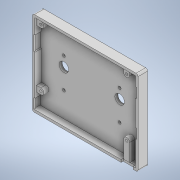
# Autodesk Inventor part: jetson_din_connector
Saved by Autodesk Inventor 2021 (Build 250183000, 183)
## iProperties
Created: 2020-10-27
Part Number: jetson_din_connector
Material: Generic
Document SubType Name: Modeling
Designer: Mateusz
Density: 1 g/cm^3
Appearance: Default
Author: Mateusz
Autodesk Inventor part; units mm, degrees
ref_plane "YZ Plane" through (0, 0, 0) normal (1, 0, 0) x (0, 1, 0)
ref_plane "XZ Plane" through (0, 0, 0) normal (0, 1, 0) x (-1, 0, 0)
ref_plane "Work Plane1" through (95.4, -17, 0) normal (0, 0, -1) x (-1, 0, 0)
sketch "Sketch1" plane through (95.4, -17, 0) normal (0, 0, -1) x (-1, 0, 0)
  line L0 (0, 79) -> (98.8, 79) projected
  line L1 (-0.6, 0.6) -> (-0.6, 78.4) projected
  line L2 (99.4, 78.4) -> (99.4, 0.6) projected
  line L3 (98.8, 0) -> (0, 0) projected
  line L4 (0, 79) -> (-0.6, 79)
  line L5 (-0.6, 79) -> (-0.6, 78.4)
  line L6 (98.8, 79) -> (99.4, 79)
  line L7 (99.4, 79) -> (99.4, 78.4)
  line L8 (98.8, 0) -> (99.4, 0)
  line L9 (99.4, 0) -> (99.4, 0.6)
  line L10 (0, 0) -> (-0.6, 0)
  line L11 (-0.6, 0.6) -> (-0.6, 0)
  circle A0 centre (9.4, 17) radius 1.45
  circle A1 centre (95.4, 17) radius 1.45
  circle A2 centre (95.4, 75) radius 1.45
  circle A3 centre (9.4, 75) radius 1.45
  line L12 (-0.6, 79) -> (-3.6, 79)
  line L13 (-3.6, 79) -> (-3.6, 0)
  line L14 (-3.6, 0) -> (-0.6, 0)
  line L15 (-3.6, 0) -> (-3.6, -3)
  line L16 (-3.6, -3) -> (99.4, -3)
  line L17 (99.4, -3) -> (102.4, -3)
  line L18 (102.4, -3) -> (102.3495, 79)
  line L19 (102.3495, 79) -> (102.3476, 82)
  line L20 (102.3476, 82) -> (-3.6, 82)
  line L21 (-3.6, 82) -> (-3.6, 79)
  dimension "d0" = 2.9
  dimension "d1" = 2.9
  dimension "d2" = 2.9
  dimension "d3" = 2.9
  dimension "d4" = 3
  dimension "d5" = 3
  dimension "d6" = 3
  dimension "d7" = 3
  constraints: 36 end point, 8 perpendicular, 7 point on line, 4 centre point, 2 horizontal, 2 parallel, 1 vertical
  measures "d0" diameter of A0
  measures "d1" diameter of A1
  measures "d2" diameter of A2
  measures "d3" diameter of A3
  measures "d4" distance of L4.end L12.end
  measures "d5" distance of L13.end L15.end
  measures "d6" distance of L16.end L17.end
  measures "d7" distance of L18.end L19.end
extrude "Extrusion1" add sketch "Sketch1" against normal blind 3
sketch "Sketch2" plane through (95.4, -17, 3) normal (0, 0, 1) x (-1, 0, 0)
  circle A0 centre (9.4, -75) radius 1.45 projected
  circle A1 centre (9.4, -75) radius 1.45
  circle A2 centre (9.4, -75) radius 3
  circle A3 centre (9.4, -17) radius 1.45 projected
  circle A4 centre (9.4, -17) radius 3
  circle A5 centre (95.4, -17) radius 1.45 projected
  circle A6 centre (95.4, -17) radius 1.45
  circle A7 centre (95.4, -17) radius 3
  circle A8 centre (95.4, -75) radius 1.45 projected
  circle A9 centre (95.4, -75) radius 3
  circle A10 centre (95.4, -75) radius 1.45
  line L0 (95.4, -78) -> (102.3501, -78)
  line L1 (102.3476, -82) -> (102.4, 3) projected
  line L2 (95.4, -72) -> (102.3501, -72)
  line L3 (102.3501, -72) -> (102.3501, -78)
  line L4 (6.4, -75) -> (6.4, -82)
  line L5 (-3.6, -82) -> (102.3476, -82) projected
  line L6 (12.4, -75) -> (12.4, -82)
  line L7 (6.4, -82) -> (12.4, -82)
  line L8 (6.4, -17) -> (6.4, 3)
  line L9 (102.4, 3) -> (-3.6, 3) projected
  line L10 (12.4, -17) -> (12.4, 3)
  line L11 (12.4, 3) -> (6.4, 3)
  line L12 (95.4, -20) -> (102.3501, -20)
  line L13 (102.3501, -20) -> (102.3501, -14)
  line L14 (102.3501, -14) -> (95.4, -14)
  point P0 (12.4, 3)
  dimension "d10" = 6
  dimension "d11" = 6
  dimension "d12" = 6
  dimension "d13" = 6
  constraints: 24 end point, 10 point on line, 8 point on circle, 7 centre point, 7 coincident, 4 parallel, 3 perpendicular, 3 tangent, 1 horizontal
  measures "d10" diameter of A2
  measures "d11" diameter of A4
  measures "d12" diameter of A7
  measures "d13" diameter of A9
extrude "Extrusion2" add sketch "Sketch2" along normal blind 5
sketch "Sketch7" plane through (95.4, -17, 3) normal (0, 0, 1) x (1, 0, 0)
  circle A0 centre (-77.3738, 24.5) radius 1.45 projected
  circle A1 centre (-21.4, 24.5) radius 1.45 projected
  circle A2 centre (-21.4, 54.5) radius 1.45 projected
  circle A3 centre (-77.3738, 54.5) radius 1.45 projected
  point P0 (-95.4, 17)
extrude "Extrusion7" cut sketch "Sketch7" against normal blind 6
sketch "Sketch8" plane through (95.4, -17, 3) normal (0, 0, 1) x (1, 0, 0)
  line L0 (-102.3476, 82) -> (3.6, 82) projected
  line L1 (-102.3476, 82) -> (-102.4, -3) projected
  line L2 (-102.3476, 82) -> (-102.4, -3)
  line L3 (-102.4, -3) -> (3.6, -3) projected
  line L4 (-102.4, -3) -> (3.6, -3)
  line L5 (3.6, -3) -> (3.6, 82)
  line L6 (3.6, 82) -> (-102.3476, 82)
  line L7 (-102.3476, 82) -> (-99.3476, 82)
  line L8 (-99.3476, 82) -> (-99.3476, -3)
  line L9 (-99.3476, -3) -> (-99.3476, 0)
  line L10 (-99.3476, 0) -> (3.6, 0)
  line L11 (3.6, -3) -> (3.6, 82) projected
  line L12 (3.6, 0) -> (0.6, 0)
  line L13 (0.6, 0) -> (0.6, 82)
  line L14 (0.6, 82) -> (0.6, 79)
  line L15 (0.6, 79) -> (-102.3495, 79)
  line L16 (-99.3476, 79) -> (-99.8476, 79)
  line L17 (-99.8476, 79) -> (-99.8476, 0)
  line L18 (-99.8476, 0) -> (-99.8476, -0.5)
  line L19 (-99.8476, -0.5) -> (0.6, -0.5)
  line L20 (0.6, -0.5) -> (1.1, -0.5)
  line L21 (1.1, -0.5) -> (1.1, 79)
  line L22 (1.1, 79) -> (1.1, 79.5)
  line L23 (1.1, 79.5) -> (-99.8476, 79.5)
  line L24 (-99.8476, 79.5) -> (-99.8476, 79)
  point P0 (-95.4, 17)
  dimension "d45" = 3
  dimension "d46" = 3
  dimension "d47" = 3
  dimension "d48" = 3
  dimension "d67" = 0.5
  dimension "d68" = 0.5
  dimension "d69" = 0.5
  dimension "d70" = 0.5
  constraints: 42 end point, 16 point on line, 9 perpendicular, 2 collinear, 2 parallel
  measures "d45" distance of L0.start L7.end
  measures "d46" distance of L8.end L9.end
  measures "d47" distance of L10.end L12.end
  measures "d48" distance of L13.end L14.end
  measures "d67" distance of L16.start L16.end
  measures "d68" distance of L17.end L18.end
  measures "d69" distance of L19.end L20.end
  measures "d70" distance of L21.end L22.end
extrude "Extrusion8" add sketch "Sketch8" along normal blind 6.57 contours L0 L8 L23 L24 L15 L1 | L0 L13 L23 L8 | L15 L17 L18 L19 L8 L3 L1 | L0 L5 L10 L21 L22 L23 L13 | L8 L19 L20 L21 L10 L5 L3
fillet "Fillet1" radius 2 4 edges at (-7, -20, 4.785) (99, -20, 4.785) (99, 65, 4.785) (-6.9476, 65, 4.785)
sketch "Sketch10" plane through (-4.9988, -20, 0) normal (0, -1, 0) x (1, 0, 0)
  line L0 (86.9988, 9.57) -> (86.9988, 13.7962) projected
  line L1 (86.9988, 13.7962) -> (98.9988, 13.7962) projected
  line L2 (98.9988, 13.7962) -> (98.9988, 9.57) projected
  line L3 (86.9988, 9.57) -> (98.9988, 9.57)
  line L4 (101.9988, 9.57) -> (0.0499, 9.57) projected
  line L5 (98.9988, 9.57) -> (98.9988, 7.57)
  line L6 (98.9988, 7.57) -> (86.9988, 7.57)
  line L7 (86.9988, 7.57) -> (86.9988, 9.57)
  point P0 (4.9988, 0)
  dimension "d72" = 2
  constraints: 8 end point, 2 perpendicular, 1 collinear, 1 point on line
  measures "d72" distance of L2.end L5.end
extrude "Extrusion9" cut sketch "Sketch10" against normal up to surface (2.5 mm away) contours L3 L5 L6 L7
sketch "Sketch11" plane through (-4.4476, 3, 3) normal (1, 0, 0) x (0, 0, -1)
  line L0 (-5, -6) -> (0, -6) projected
  line L1 (-5, 0) -> (-5, -6) projected
  line L2 (0, 0) -> (-5, 0) projected
  line L3 (0, 52) -> (0, 0) projected
  line L4 (-5, 52) -> (0, 52) projected
  line L5 (-5, 58) -> (-5, 52) projected
  line L6 (0, 58) -> (-5, 58) projected
  line L7 (0, 59.5) -> (0, 58) projected
  line L8 (0, 59.5) -> (-6.57, 59.5) projected
  line L9 (-6.57, -20.5) -> (-6.57, 59.5) projected
  line L10 (0, -20.5) -> (-6.57, -20.5) projected
  line L11 (0, -6) -> (0, -20.5) projected
  line L12 (-6.57, 60.0012) -> (-6.57, -20.9988) projected
  line L13 (-6.57, 19.5012) -> (0, 19.5012)
  line L14 (0, 52) -> (0, 0) projected
  line L15 (-6.57, 59.5) -> (-6.57, 44.5)
  line L16 (-6.57, 44.5) -> (0, 44.5)
  line L17 (0, -20.5) -> (0, 59.5) projected
  line L18 (-6.57, 44.5) -> (0, 44.5)
  line L19 (0, 44.5) -> (0, 29.5)
  line L20 (0, 29.5) -> (-6.57, 29.5)
  line L21 (-6.57, 29.5) -> (-6.57, 44.5)
  line L22 (-4.57, -20.5) -> (-6.57, -20.5) projected
  line L23 (-6.57, -20.5) -> (-6.57, 4.5)
  line L24 (-6.57, 4.5) -> (0, 4.5)
  line L25 (0, -3) -> (0, -20.5) projected
  line L26 (-6.57, -20.5) -> (0, -20.5)
  line L27 (0, -20.5) -> (0, -10.5)
  line L28 (0, -10.5) -> (-6.57, -10.5)
  line L29 (-6.57, -10.5) -> (-6.57, -20.5)
  line L30 (-6.57, -20.5) -> (-4.57, -20.5)
  line L31 (-4.57, -20.5) -> (-4.57, -10.5)
  line L32 (-6.57, 29.5) -> (-4.57, 29.5)
  line L33 (-4.57, 29.5) -> (-4.57, 44.5)
  point P0 (3, -3)
  point P1 (-4.57, 44.5)
  dimension "d75" = 15
  dimension "d76" = 15
  dimension "d77" = 25
  dimension "d78" = 10
  dimension "d79" = 2
  dimension "d80" = 2
  constraints: 34 end point, 8 point on line, 5 perpendicular, 4 parallel, 3 horizontal, 1 collinear, 1 midpoint, 4 other
  measures "d75" distance of L8.end L15.end
  measures "d76" distance of L18.end L19.end
  measures "d77" distance of L9.start L23.end
  measures "d78" distance of L27.end L26.end
  measures "d79" distance of L9.start L22.start
  measures "d80" distance of L20.end L32.end
extrude "Extrusion10" cut sketch "Sketch11" against normal blind 1.5 contours L11 L10 L31 L28 | L20 L33 L16 L3
sketch "Sketch12" plane through (96.5, -17.5, 3) normal (-1, 0, 0) x (0, 0, 1)
  line L0 (0, 0) -> (0, 80) projected
  line L1 (0, 0) -> (6.57, 0) projected
  line L2 (6.57, 80) -> (6.57, 0) projected
  line L3 (0, 80) -> (6.57, 80) projected
  line L4 (6.57, 80.5012) -> (6.57, -0.4988) projected
  line L5 (6.57, 80.5012) -> (6.57, 70.5012)
  line L6 (0, 65) -> (0, 50) projected
  line L7 (6.57, 70.5012) -> (0, 70.5012)
  line L8 (0, 70.5012) -> (0, 60.5012)
  line L9 (0, 60.5012) -> (6.57, 60.5012)
  line L10 (6.57, 60.5012) -> (6.57, 70.5012)
  line L11 (0, 17.5) -> (0, 0) projected
  line L12 (0, 0) -> (0, 25)
  line L13 (0, 50) -> (0, 20.5) projected
  line L14 (0, 25) -> (6.57, 25)
  line L15 (6.57, 25) -> (6.57, 35)
  line L16 (6.57, 35) -> (0, 35)
  line L17 (0, 35) -> (0, 25)
  line L18 (6.57, 35) -> (4.57, 35)
  line L19 (4.57, 35) -> (4.57, 25)
  line L20 (6.57, 70.5012) -> (4.57, 70.5012)
  line L21 (4.57, 70.5012) -> (4.57, 60.5012)
  line L22 (4.57, 50) -> (4.57, 65) projected
  point P0 (-3, 17.5)
  dimension "d83" = 10
  dimension "d84" = 10
  dimension "d85" = 25
  dimension "d86" = 10
  dimension "d87" = 2
  dimension "d88" = 2
  constraints: 28 end point, 9 point on line, 4 parallel, 3 perpendicular, 2 horizontal
  measures "d83" distance of L4.start L5.end
  measures "d84" distance of L8.end L7.end
  measures "d85" distance of L0.start L12.end
  measures "d86" distance of L15.end L14.end
  measures "d87" distance of L15.end L18.end
  measures "d88" distance of L5.end L20.end
extrude "Extrusion11" cut sketch "Sketch12" against normal blind 1.5 contours L0 L16 L19 L14 | L9 L0 L7 L21
sketch "Sketch15" plane through (95.4, -17, 9.57) normal (0, 0, 1) x (1, 0, 0)
  line L0 (-99.8476, 64.5) -> (-101.3476, 64.5) projected
  line L1 (-99.8476, 49.5) -> (-99.8476, 64.5) projected
  line L2 (-99.8476, 64.5) -> (-99.8476, 49.5)
  line L3 (-99.8476, 49.5) -> (-100.8476, 49.5)
  line L4 (-100.8476, 49.5) -> (-100.8476, 64.5)
  line L5 (-99.8476, -0.5) -> (-99.8476, 9.5) projected
  line L6 (-99.8476, 9.5) -> (-100.8476, 9.5)
  line L7 (-100.8476, 9.5) -> (-100.8476, -0.5)
  line L8 (-100.8476, -0.5) -> (-99.8476, -0.5)
  line L9 (1.1, 34.5) -> (2.6, 34.5) projected
  line L10 (1.1, 34.5) -> (2.1, 34.5)
  line L11 (2.1, 34.5) -> (2.1, 24.5)
  line L12 (1.1, 24.5) -> (2.6, 24.5) projected
  line L13 (1.1, 24.5) -> (1.1, 34.5)
  line L14 (1.1, 79.5) -> (1.1, -0.5) projected
  line L15 (1.1, 60.0012) -> (2.6, 60.0012) projected
  line L16 (1.1, 70.0012) -> (2.6, 70.0012) projected
  line L17 (1.1, 60.0012) -> (1.1, 70.0012)
  line L18 (1.1, 70.0012) -> (2.1, 70.0012)
  line L19 (2.1, 70.0012) -> (2.1, 60.0012)
  point P0 (-95.4, 17)
  point P1 (2.1, 60.0012)
  dimension "d95" = 1
  dimension "d96" = 1
  dimension "d97" = 1
  dimension "d98" = 1
  constraints: 24 end point, 6 perpendicular, 3 point on line, 2 collinear, 1 horizontal, 1 vertical
  measures "d95" distance of L1.start L3.end
  measures "d96" distance of L5.end L6.end
  measures "d97" distance of L9.start L10.end
  measures "d98" distance of L16.start L18.end
extrude "Extrusion14" cut sketch "Sketch15" against normal blind 2
sketch "Sketch16" plane through (95.4, -17, 8) normal (0, 0, 1) x (1, 0, 0)
  circle A0 centre (-95.4, 17) radius 1.2
  circle A1 centre (-9.4, 17) radius 1.45 projected
  circle A2 centre (-9.4, 17) radius 1.2
  circle A3 centre (-9.4, 75) radius 1.45 projected
  circle A4 centre (-9.4, 75) radius 1.2
  circle A5 centre (-95.4, 75) radius 1.45 projected
  circle A6 centre (-95.4, 75) radius 1.2
  circle A7 centre (-9.4, 75) radius 1.45 projected
  circle A8 centre (-95.4, 17) radius 1.45 projected
  dimension "d101" = 2.4
  dimension "d102" = 2.4
  dimension "d103" = 2.4
  dimension "d104" = 2.4
  constraints: 4 centre point, 4 coincident
  measures "d101" diameter of A0
  measures "d102" diameter of A2
  measures "d103" diameter of A4
  measures "d104" diameter of A6
extrude "Extrusion15" add sketch "Sketch16" against normal up to surface (8 mm away)
sketch "Sketch17" plane through (95.4, -17, 3) normal (0, 0, 1) x (1, 0, 0)
  circle A0 centre (-77.3738, 54.5) radius 1.45 projected
  circle A1 centre (-21.4, 54.5) radius 1.45 projected
  circle A2 centre (-77.3738, 44.568) radius 4.767
  line L0 (-21.4, 54.5) -> (-21.4, 44.568)
  circle A3 centre (-21.4, 44.568) radius 4.767
  point P0 (-95.4, 17)
  dimension "d108" = 9.534
  constraints: 2 centre point, 2 end point, 1 coincident, 1 vertical
  measures "d108" diameter of A2
extrude "Extrusion16" cut sketch "Sketch17" against normal up to surface (3 mm away) contours A2 | A3
equation "\"d43\" = d42"
equation "\"d42\" = 6"
body "Solid924"
